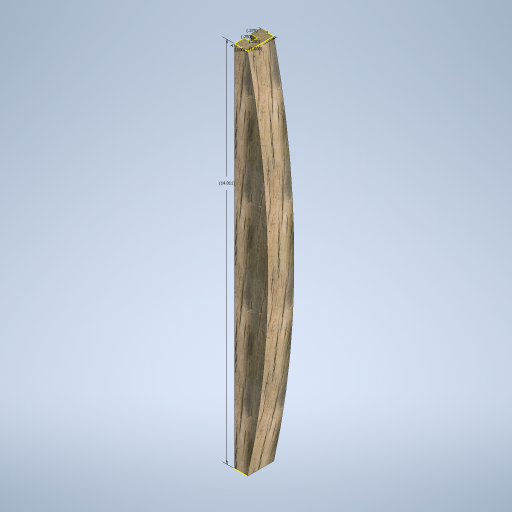
# Autodesk Inventor part: sidestrip_Ocampo
Saved by Autodesk Inventor 2023 (Build 270158000, 158)
## iProperties
Created: 2025-03-24
Part Number: sidestrip_Ocampo
Material: Generic
Document SubType Name: Modeling
Designer: 1244275
Density: 1 g/cm^3
Appearance: Default
Author: 1244275
Autodesk Inventor part; units mm, degrees
ref_plane "YZ Plane" through (0, 0, 0) normal (1, 0, 0) x (0, 1, 0)
ref_plane "XZ Plane" through (0, 0, 0) normal (0, 1, 0) x (-1, 0, 0)
ref_plane "XY Plane" through (0, 0, 0) normal (0, 0, 1) x (1, 0, 0)
sketch "Sketch1" plane through (0, 0, 0) normal (0, 0, 1) x (1, 0, 0)
  line L0 (0, 0) -> (12.7, 0)
  line L1 (0, 0) -> (0, 355.8819)
  line L2 (0, 355.8819) -> (12.7, 355.8819)
  arc A0 (12.7, 0) -> (12.7, 355.8819) centre (-782.8431, 177.941) ccw
  dimension "d0" = 12.7
  dimension "d1" = 355.8819
  dimension "d2" = 12.7
  constraints: 6 end point, 2 horizontal, 2 point on circle, 1 centre point, 1 vertical
  measures "d0" distance of L0.start L0.end
  measures "d1" distance of L0.start L1.end
  measures "d2" distance of L1.end L2.end
extrude "Extrusion1" add sketch "Sketch1" along normal blind 25.4
sketch "Sketch2" plane through (0, 0, 0) normal (-1, 0, 0) x (0, 0, 1)
  line L0 (0, 0) -> (12.7, 0)
  line L1 (0, 0) -> (25.4, 0) projected
  line L2 (12.7, 355.8819) -> (9.525, 355.8819)
  line L3 (9.525, 355.8819) -> (9.525, 0)
  line L4 (9.525, 0) -> (15.875, 0)
  line L5 (15.875, 0) -> (15.875, 355.8819)
  line L6 (9.525, 355.8819) -> (15.875, 355.8819)
  line L7 (9.525, 0) -> (15.875, 0)
  dimension "d5" = 12.7
  dimension "d6" = 3.175
  dimension "d7" = 6.35
  constraints: 14 end point, 2 perpendicular, 2 point on line, 1 collinear, 1 midpoint
  measures "d5" distance of L0.start L0.end
  measures "d6" distance of L2.start L2.end
  measures "d7" distance of L3.end L4.end
extrude "Extrusion2" cut sketch "Sketch2" against normal blind 6.35
sketch "Sketch3" plane through (0, 355.8819, 0) normal (0, 1, 0) x (1, 0, 0)
  line L0 (12.7, -25.4) -> (0, -25.4) projected
  line L1 (12.7, 0) -> (0, 0) projected
  line L2 (0, -9.525) -> (6.35, -9.525) projected
  line L3 (6.35, -15.875) -> (0, -15.875) projected
  line L4 (6.35, -9.525) -> (6.35, -15.875) projected
  line L5 (0, -15.875) -> (0, -25.4) projected
  line L6 (12.7, 0) -> (12.7, -25.4) projected
  point P0 (6.35, 0)
  dimension "d10" = 25.4
  dimension "d11" = 9.525
  dimension "d12" = 6.35
  dimension "d13" = 6.35
  dimension "d14" = 12.7
  constraints: 1 midpoint
  measures "d10" distance between parallel lines of L0 L1
  measures "d11" distance from line of L2 point (6.35, 0)
  measures "d12" distance between parallel lines of L3 L2
  measures "d13" distance from line of L3.end L4
  measures "d14" distance between parallel lines of L5 L6
sketch "Sketch4" plane through (0, 0, 25.4) normal (0, 0, 1) x (1, 0, 0)
  line L0 (12.7, 355.8819) -> (0, 355.8819) projected
  line L1 (0, 0) -> (12.7, 0) projected
  dimension "d15" = 355.8819
  measures "d15" distance between parallel lines of L0 L1
body "Solid1"
